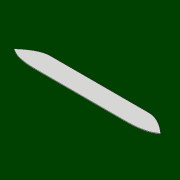
# Autodesk Inventor part: Part4
Saved by Autodesk Inventor 2018 (Build 220112000, 112)
## iProperties
Created: 2021-12-12
Part Number: Part4
Material: 一般
Document SubType Name: Modeling
Designer: gisen
Density: 1 g/cm^3
Appearance: 既定
Author: gisen
Autodesk Inventor part; units mm, degrees
ref_plane "YZ Plane" through (0, 0, 0) normal (1, 0, 0) x (0, 1, 0)
ref_plane "XZ Plane" through (0, 0, 0) normal (0, 1, 0) x (-1, 0, 0)
ref_plane "XY Plane" through (0, 0, 0) normal (0, 0, 1) x (1, 0, 0)
sketch "スケッチ1" plane through (0, 0, 0) normal (0, 0, 1) x (1, 0, 0)
  line L0 (352.3119, 260.3111) -> (356.9762, 260.4005)
  line L1 (356.9762, 260.4005) -> (361.3502, 260.6571)
  line L2 (361.3502, 260.6571) -> (365.41, 261.0613)
  line L3 (365.41, 261.0613) -> (369.1508, 261.5942)
  line L4 (369.1508, 261.5942) -> (372.5686, 262.2371)
  line L5 (372.5686, 262.2371) -> (375.6597, 262.9714)
  line L6 (375.6597, 262.9714) -> (378.4213, 263.7798)
  line L7 (378.4213, 263.7798) -> (380.852, 264.6459)
  line L8 (380.852, 264.6459) -> (382.9528, 265.5562)
  line L9 (382.9528, 265.5562) -> (384.6784, 266.4765)
  line L10 (384.6784, 266.4765) -> (389.6023, 269.4159)
  line L11 (389.6023, 269.4159) -> (385.1952, 273.0342)
  line L12 (385.1952, 273.0342) -> (382.9844, 274.7929)
  line L13 (382.9844, 274.7929) -> (380.7625, 276.4426)
  line L14 (380.7625, 276.4426) -> (378.5463, 277.9704)
  line L15 (378.5463, 277.9704) -> (376.34, 279.3736)
  line L16 (376.34, 279.3736) -> (374.1475, 280.6496)
  line L17 (374.1475, 280.6496) -> (371.9725, 281.7954)
  line L18 (371.9725, 281.7954) -> (369.8187, 282.8081)
  line L19 (369.8187, 282.8081) -> (367.6896, 283.6845)
  line L20 (367.6896, 283.6845) -> (365.5886, 284.4211)
  line L21 (365.5886, 284.4211) -> (363.5401, 285.008)
  line L22 (363.5401, 285.008) -> (362.8461, 285.1759)
  line L23 (362.8461, 285.1759) -> (362.1766, 285.3224)
  line L24 (362.1766, 285.3224) -> (361.5121, 285.4522)
  line L25 (361.5121, 285.4522) -> (360.8528, 285.5651)
  line L26 (360.8528, 285.5651) -> (360.199, 285.6611)
  line L27 (360.199, 285.6611) -> (359.551, 285.74)
  line L28 (359.551, 285.74) -> (358.9089, 285.8017)
  line L29 (358.9089, 285.8017) -> (358.2731, 285.8459)
  line L30 (358.2731, 285.8459) -> (357.6439, 285.8726)
  line L31 (357.6439, 285.8726) -> (357.0361, 285.8814)
  line L32 (357.0361, 285.8814) -> (221.1491, 285.8814)
  line L33 (221.1491, 285.8814) -> (220.5415, 285.8726)
  line L34 (220.5415, 285.8726) -> (219.9125, 285.8459)
  line L35 (219.9125, 285.8459) -> (219.2769, 285.8017)
  line L36 (219.2769, 285.8017) -> (218.6349, 285.74)
  line L37 (218.6349, 285.74) -> (217.9869, 285.6611)
  line L38 (217.9869, 285.6611) -> (217.3331, 285.5651)
  line L39 (217.3331, 285.5651) -> (216.6737, 285.4522)
  line L40 (216.6737, 285.4522) -> (216.009, 285.3224)
  line L41 (216.009, 285.3224) -> (215.3393, 285.176)
  line L42 (215.3393, 285.176) -> (214.6449, 285.0081)
  line L43 (214.6449, 285.0081) -> (212.5963, 284.4211)
  line L44 (212.5963, 284.4211) -> (210.4955, 283.6844)
  line L45 (210.4955, 283.6844) -> (208.3666, 282.8081)
  line L46 (208.3666, 282.8081) -> (206.213, 281.7953)
  line L47 (206.213, 281.7953) -> (204.0383, 280.6496)
  line L48 (204.0383, 280.6496) -> (201.8458, 279.3736)
  line L49 (201.8458, 279.3736) -> (199.6395, 277.9704)
  line L50 (199.6395, 277.9704) -> (197.4231, 276.4427)
  line L51 (197.4231, 276.4427) -> (195.2007, 274.7931)
  line L52 (195.2007, 274.7931) -> (192.9885, 273.0339)
  line L53 (192.9885, 273.0339) -> (188.5872, 269.4157)
  line L54 (188.5872, 269.4157) -> (193.5061, 266.4766)
  line L55 (193.5061, 266.4766) -> (195.2328, 265.5561)
  line L56 (195.2328, 265.5561) -> (197.3339, 264.6458)
  line L57 (197.3339, 264.6458) -> (199.7649, 263.7797)
  line L58 (199.7649, 263.7797) -> (202.5267, 262.9714)
  line L59 (202.5267, 262.9714) -> (205.6178, 262.237)
  line L60 (205.6178, 262.237) -> (209.0357, 261.5942)
  line L61 (209.0357, 261.5942) -> (212.7765, 261.0613)
  line L62 (212.7765, 261.0613) -> (216.8361, 260.6571)
  line L63 (216.8361, 260.6571) -> (221.2101, 260.4005)
  line L64 (221.2101, 260.4005) -> (225.8743, 260.3111)
  line L65 (225.8743, 260.3111) -> (352.3119, 260.3111)
  point P0 (0, 0)
  constraints: 132 end point
extrude "押し出し1" add sketch "スケッチ1" along normal blind 1
